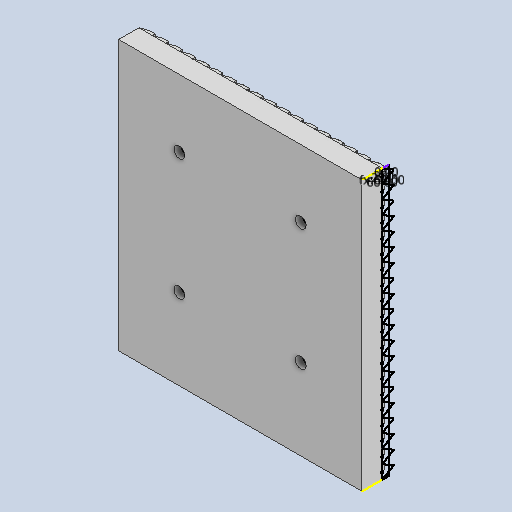
# Autodesk Inventor part: Gripper plate v1
Saved by Autodesk Inventor 2023 (Build 270158000, 158)
## iProperties
Created: 2023-02-07
Part Number: Gripper plate v1
Material: Generic
Document SubType Name: Modeling
Designer: Gabriel - T3 CAD
Density: 1 g/cm^3
Appearance: Default
Author: Gabriel - T3 CAD
Autodesk Inventor part; units mm, degrees
ref_plane "YZ Plane" through (0, 0, 0) normal (1, 0, 0) x (0, 1, 0)
ref_plane "XZ Plane" through (0, 0, 0) normal (0, 1, 0) x (-1, 0, 0)
ref_plane "XY Plane" through (0, 0, 0) normal (0, 0, 1) x (1, 0, 0)
sketch "Sketch1" plane through (0, 0, 0) normal (0, 0, 1) x (1, 0, 0)
  line L0 (0, 0) -> (114.3, 0)
  line L1 (114.3, 0) -> (114.3, 127)
  line L2 (114.3, 127) -> (0, 127)
  line L3 (0, 127) -> (0, 0)
  circle A0 centre (28.575, 38.1) radius 2.5797
  circle A1 centre (85.725, 38.1) radius 2.5797
  circle A2 centre (28.575, 95.25) radius 2.5797
  circle A3 centre (85.725, 95.25) radius 2.5797
  circle A4 centre (28.575, 38.1) radius 5.08
  circle A5 centre (85.725, 38.1) radius 5.08
  circle A6 centre (28.575, 95.25) radius 5.08
  circle A7 centre (85.725, 95.25) radius 5.08
  dimension "d0" = 114.3
  dimension "d1" = 127
  dimension "d2" = 28.575
  dimension "d3" = 38.1
  dimension "d4" = 5.1594
  dimension "d7" = 57.15
  dimension "d10" = 57.15
  dimension "d56" = 10.16
  dimension "d59" = 57.15
  dimension "d62" = 57.15
  constraints: 8 centre point, 8 end point, 4 coincident, 3 horizontal, 2 parallel, 2 vertical, 1 perpendicular, 15 other
  measures "d0" distance of L2.end L1.end
  measures "d1" distance of L1.end L0.end
  measures "d2" distance from line of L3 A0.centre
  measures "d3" distance from line of L0 A0.centre
  measures "d4" diameter of A0
  measures "d7" distance of A0.centre A1.centre
  measures "d10" distance of A0.centre A2.centre
  measures "d56" diameter of A4
  measures "d59" distance of A0.centre point (85.725, 38.1)
  measures "d62" distance of A0.centre point (28.575, 95.25)
extrude "Extrusion1" add sketch "Sketch1" along normal blind 12.7 contours L3 L2 L1 L0 | A4 | A5 | A6 | A7
sketch "Sketch2" plane through (114.3, 0, 0) normal (1, 0, 0) x (0, 0, -1)
  line L0 (-3.175, 127) -> (2.3243, 123.825)
  line L1 (2.3243, 123.825) -> (-3.175, 120.65)
  line L2 (-3.175, 120.65) -> (-3.175, 127)
  line L3 (0, 0) -> (0, 127) projected
  line L4 (0, 127) -> (-12.7, 127) projected
  line L5 (-3.175, 120.65) -> (2.3243, 117.475)
  line L6 (2.3243, 117.475) -> (-3.175, 114.3)
  line L7 (-3.175, 114.3) -> (-3.175, 120.65)
  line L8 (-3.175, 114.3) -> (2.3243, 111.125)
  line L9 (2.3243, 111.125) -> (-3.175, 107.95)
  line L10 (-3.175, 107.95) -> (-3.175, 114.3)
  line L11 (-3.175, 107.95) -> (2.3243, 104.775)
  line L12 (2.3243, 104.775) -> (-3.175, 101.6)
  line L13 (-3.175, 101.6) -> (-3.175, 107.95)
  line L14 (-3.175, 101.6) -> (2.3243, 98.425)
  line L15 (2.3243, 98.425) -> (-3.175, 95.25)
  line L16 (-3.175, 95.25) -> (-3.175, 101.6)
  line L17 (-3.175, 95.25) -> (2.3243, 92.075)
  line L18 (2.3243, 92.075) -> (-3.175, 88.9)
  line L19 (-3.175, 88.9) -> (-3.175, 95.25)
  line L20 (-3.175, 88.9) -> (2.3243, 85.725)
  line L21 (2.3243, 85.725) -> (-3.175, 82.55)
  line L22 (-3.175, 82.55) -> (-3.175, 88.9)
  line L23 (-3.175, 82.55) -> (2.3243, 79.375)
  line L24 (2.3243, 79.375) -> (-3.175, 76.2)
  line L25 (-3.175, 76.2) -> (-3.175, 82.55)
  line L26 (-3.175, 76.2) -> (2.3243, 73.025)
  line L27 (2.3243, 73.025) -> (-3.175, 69.85)
  line L28 (-3.175, 69.85) -> (-3.175, 76.2)
  line L29 (-3.175, 69.85) -> (2.3243, 66.675)
  line L30 (2.3243, 66.675) -> (-3.175, 63.5)
  line L31 (-3.175, 63.5) -> (-3.175, 69.85)
  line L32 (-3.175, 63.5) -> (2.3243, 60.325)
  line L33 (2.3243, 60.325) -> (-3.175, 57.15)
  line L34 (-3.175, 57.15) -> (-3.175, 63.5)
  line L35 (-3.175, 57.15) -> (2.3243, 53.975)
  line L36 (2.3243, 53.975) -> (-3.175, 50.8)
  line L37 (-3.175, 50.8) -> (-3.175, 57.15)
  line L38 (-3.175, 50.8) -> (2.3243, 47.625)
  line L39 (2.3243, 47.625) -> (-3.175, 44.45)
  line L40 (-3.175, 44.45) -> (-3.175, 50.8)
  line L41 (-3.175, 44.45) -> (2.3243, 41.275)
  line L42 (2.3243, 41.275) -> (-3.175, 38.1)
  line L43 (-3.175, 38.1) -> (-3.175, 44.45)
  line L44 (-3.175, 38.1) -> (2.3243, 34.925)
  line L45 (2.3243, 34.925) -> (-3.175, 31.75)
  line L46 (-3.175, 31.75) -> (-3.175, 38.1)
  line L47 (-3.175, 31.75) -> (2.3243, 28.575)
  line L48 (2.3243, 28.575) -> (-3.175, 25.4)
  line L49 (-3.175, 25.4) -> (-3.175, 31.75)
  line L50 (-3.175, 25.4) -> (2.3243, 22.225)
  line L51 (2.3243, 22.225) -> (-3.175, 19.05)
  line L52 (-3.175, 19.05) -> (-3.175, 25.4)
  line L53 (-3.175, 19.05) -> (2.3243, 15.875)
  line L54 (2.3243, 15.875) -> (-3.175, 12.7)
  line L55 (-3.175, 12.7) -> (-3.175, 19.05)
  line L56 (-3.175, 12.7) -> (2.3243, 9.525)
  line L57 (2.3243, 9.525) -> (-3.175, 6.35)
  line L58 (-3.175, 6.35) -> (-3.175, 12.7)
  line L59 (-3.175, 6.35) -> (2.3243, 3.175)
  line L60 (2.3243, 3.175) -> (-3.175, 0)
  line L61 (-3.175, 0) -> (-3.175, 6.35)
  line L62 (0, 0) -> (-12.7, 0) projected
  line L63 (-3.175, 0) -> (0, 0)
  line L64 (0, 0) -> (0, 127)
  line L65 (0, 127) -> (-3.175, 127)
  line L66 (-3.175, 127) -> (-3.175, 0)
  point P0 (-3.175, 123.825)
  point P1 (-3.175, 117.475)
  point P2 (-3.175, 111.125)
  point P3 (-3.175, 104.775)
  point P4 (-3.175, 98.425)
  point P5 (-3.175, 92.075)
  point P6 (-3.175, 85.725)
  point P7 (-3.175, 79.375)
  point P8 (-3.175, 73.025)
  point P9 (-3.175, 66.675)
  point P10 (-3.175, 60.325)
  point P11 (-3.175, 53.975)
  point P12 (-3.175, 47.625)
  point P13 (-3.175, 41.275)
  point P14 (-3.175, 34.925)
  point P15 (-3.175, 28.575)
  point P16 (-3.175, 22.225)
  point P17 (-3.175, 15.875)
  point P18 (-3.175, 9.525)
  point P19 (-3.175, 3.175)
  point P20 (0, 1.8331)
  point P21 (0, 125.1669)
  point P22 (0, 4.5169)
  point P23 (0, 8.1831)
  point P24 (0, 118.8169)
  point P25 (0, 122.4831)
  dimension "d15" = 60
  dimension "d16" = 60
  dimension "d17" = 0
  dimension "d18" = 6.35
  dimension "d19" = 3.175
  dimension "d22" = 6.35
  constraints: 128 end point, 3 point on line, 2 parallel, 1 collinear, 1 midpoint, 1 perpendicular, 1 vertical, 133 other
  measures "d15" angle of L2 L1
  measures "d16" angle of L2 L0
  measures "d17" angle of L3 L2
  measures "d18" distance of L1.end L0.start
  measures "d19" distance from line of L3 point (-3.175, 123.825)
  measures "d22" distance of L0.start L5.start
extrude "Extrusion2" cut sketch "Sketch2" against normal through all contours L1 L3 L5
pattern_linear "Rectangular Pattern1" count 25 spacing 6.35 along (0, -1, 0) count 2 spacing 25.4 along (0, 1, 0) of "Extrusion2"
sketch "Sketch3" plane through (0, 127, 12.7) normal (0, 1, 0) x (1, 0, 0)
  line L0 (0, 9.525) -> (3.175, 15.0243)
  line L1 (3.175, 15.0243) -> (6.35, 9.525)
  line L2 (6.35, 9.525) -> (0, 9.525)
  line L3 (0, 12.7) -> (0, 9.525) projected
  line L4 (0, 12.7) -> (114.3, 12.7) projected
  line L5 (6.35, 9.525) -> (9.525, 15.0243)
  line L6 (9.525, 15.0243) -> (12.7, 9.525)
  line L7 (12.7, 9.525) -> (6.35, 9.525)
  line L8 (114.3, 12.7) -> (0, 12.7) projected
  line L9 (4.5169, 12.7) -> (8.1831, 12.7)
  point P0 (8.1831, 12.7)
  dimension "d37" = 60
  dimension "d38" = 60
  dimension "d39" = 6.35
  dimension "d40" = 3.175
  dimension "d43" = 6.35
  constraints: 14 end point, 5 point on line, 1 horizontal, 1 perpendicular, 6 other
  measures "d37" angle of L0 L2
  measures "d38" angle of L1 L2
  measures "d39" distance of L1.end L0.start
  measures "d40" distance between parallel lines of L4 L2
  measures "d43" distance of L0.start L5.start
extrude "Extrusion4" cut sketch "Sketch3" against normal through all contours L1 L4 L5
pattern_linear "Rectangular Pattern2" count 25 spacing 6.35 along (1, 0, 0) count 2 spacing 6.35 along (-1, 0, 0) of "Extrusion4"
extrude "Extrusion5" cut sketch "Sketch1" along normal blind 9.525 contours A0 | A1 | A2 | A3 | A4 | A5 | A6 | A7
equation "\"d59\" = d7"
equation "\"d62\" = d10"
equation "\"d16\" = d15"
equation "\"d38\" = d37"
body "Solid1"
